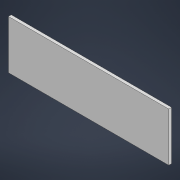
# Autodesk Inventor part: goalPanelFrontLower
Saved by Autodesk Inventor 2021 (Build 250183000, 183)
## iProperties
Created: 2021-11-25
Part Number: goalPanelFrontLower
Material: Generic
Document SubType Name: Modeling
Designer: jo_ki
Density: 1 g/cm^3
Appearance: Default
Author: jo_ki
Autodesk Inventor part; units mm, degrees
ref_plane "YZ Plane" through (0, 0, 0) normal (1, 0, 0) x (0, 1, 0)
ref_plane "XZ Plane" through (0, 0, 0) normal (0, 1, 0) x (-1, 0, 0)
ref_plane "XY Plane" through (0, 0, 0) normal (0, 0, 1) x (1, 0, 0)
sketch "Sketch1" plane through (0, 0, 0) normal (0, 0, 1) x (1, 0, 0)
  line L0 (-112, -34) -> (112, -34)
  line L1 (112, -34) -> (112, 34)
  line L2 (112, 34) -> (-112, 34)
  line L3 (-112, 34) -> (-112, -34)
  line L4 (-112, -34) -> (112, 34) construction
  line L5 (112, -34) -> (-112, 34) construction
  point P0 (0, 0)
  dimension "d0" = 224
  dimension "d2" = 68
  constraints: 12 end point, 2 midpoint, 2 parallel, 1 horizontal, 1 perpendicular
  measures "d0" distance of L1.end L2.end
  measures "d2" distance of L0.end L1.end
derived "Mastersketch.ipt"
extrude "Extrusion1" add sketch "Sketch1" along normal mid plane 4
equation "\"d0\" = goal_width"
equation "\"d2\" = goalCollector_depth"
equation "\"d3\" = goalPanel_thickness"
equation "\"goal_width\" = 224"
equation "\"goalCollector_depth\" = 68"
equation "\"goalPanel_thickness\" = 4"
body "Solid1"
